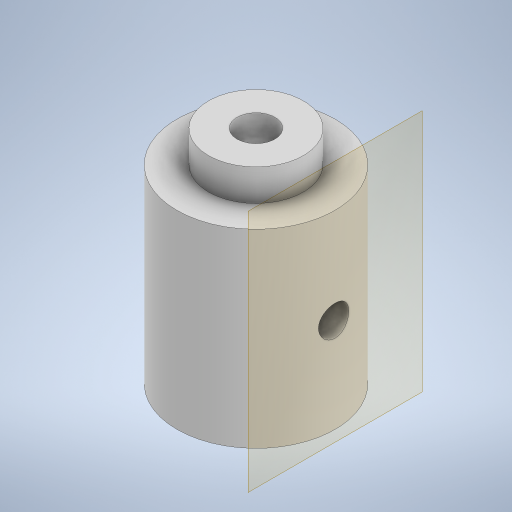
# Autodesk Inventor part: StuurPotentiometerConnector2.0
Saved by Autodesk Inventor 2024 (Build 280153000, 153)
## iProperties
Created: 2023-10-09
Part Number: StuurPotentiometerConnector2.0
Material: Generic
Document SubType Name: Modeling
Designer: Gibi500
Density: 1 g/cm^3
Appearance: Default
Author: Gibi500
## iProperties of the stored document StuurPotentiometerConnector2.0_3DPrint.ipt
Created: 2023-10-09
Part Number: StuurPotentiometerConnector2.0_3DPrint
Material: Generic
Document SubType Name: Modeling
Designer: Gibi500
Density: 1 g/cm^3
Appearance: Default
Author: Gibi500
Autodesk Inventor part; units mm, degrees
ref_plane "XZ Plane" through (0, 0, 0) normal (0, 1, 0) x (-1, 0, 0)
ref_plane "XY Plane" through (0, 0, 0) normal (0, 0, 1) x (1, 0, 0)
sketch "Sketch1" plane through (0, 0, 0) normal (1, 0, 0) x (0, 1, 0)
  line L0 (0, 0) -> (50, 0)
  line L1 (0, 5.25) -> (0, 12.5)
  line L2 (0, 12.5) -> (30, 12.5)
  line L3 (30, 12.5) -> (30, 7.5)
  line L4 (30, 7.5) -> (35, 7.5)
  line L5 (35, 7.5) -> (35, 3)
  line L6 (35, 3) -> (30, 2.5)
  line L7 (30, 2.5) -> (30, 0)
  line L8 (28, 0) -> (28, 5.25)
  line L9 (28, 5.25) -> (0, 5.25)
  line L10 (0, -2.5) -> (0, 15) projected
  dimension "d0" = 50
  dimension "d2" = 25
  dimension "d3" = 10.5
  dimension "d4" = 5
  dimension "d5" = 6
  dimension "d6" = 15
  dimension "d7" = 30
  dimension "d8" = 35
  dimension "d9" = 28
  constraints: 20 end point, 5 perpendicular, 5 point on line, 2 vertical, 1 collinear, 1 horizontal
  measures "d0" distance of L0.start L0.end
  measures "d2" diameter of L2 L0
  measures "d3" diameter of L9 L0
  measures "d4" diameter of L6.end L0
  measures "d5" diameter of L5.end L0
  measures "d6" diameter of L4 L0
  measures "d7" distance from line of L0.start L3
  measures "d8" distance from line of L0.start L5
  measures "d9" distance from line of L0.start L8
revolve "Revolution1" add sketch "Sketch1" angle 360 about axis through (0, 0, 0) along (0, 1, 0) contours L8 L9 L1 L2 L3 L4 L5 L6 L7 L0
ref_plane "Work Plane1" through (12.5, 15, 0) normal (1, 0, 0) x (0, 1, 0)
sketch "Sketch2" plane through (12.5, 15, 0) normal (1, 0, 0) x (0, 1, 0)
  line L0 (-15, 0) -> (-0.1, 0)
  circle A0 centre (-0.1, 0) radius 2.4
  dimension "d11" = 14.9
  dimension "d12" = 4.8
  constraints: 2 end point, 1 centre point, 1 coincident, 1 horizontal
  measures "d11" distance of L0.start L0.end
  measures "d12" diameter of A0
extrude "Extrusion1" cut sketch "Sketch2" against normal through all
body "Solid1"
